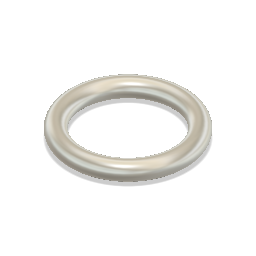
Note (Autodesk Fusion 360 design; units mm, degrees)
Autodesk Fusion 360 part; units mm, degrees
torus "TorusPrimitive1" add centre line diameter 304.8 section diameter 50.8 placed x (1, 0, 0) y (0, 0, -1) z (0, 1, 0) at (0, 0, 0) in component "Note"
component "Note" placed x (1, 0, 0) y (0, 1, 0) z (0, 0, 1) at (0, 0, 0)
